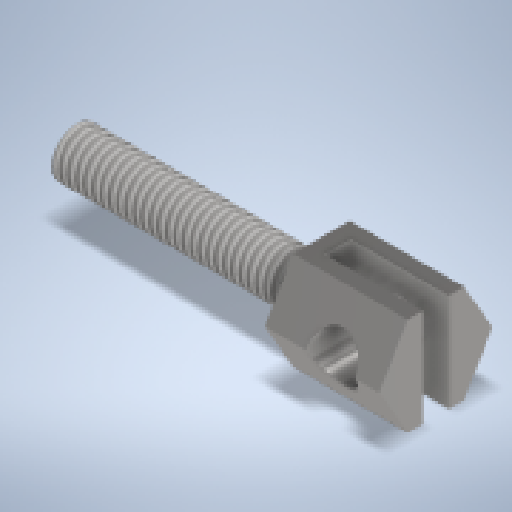
# Autodesk Inventor part: CompressionRollerArmActuatorScrew
Saved by Autodesk Inventor 2025 (Build 290162000, 162)
## iProperties
Created: 2024-08-19
Part Number: CompressionRollerArmActuatorScrew
Material: Steel, Alloy
Document SubType Name: Modeling
Designer: hello
Density: 7.73 g/cm^3
Appearance: Semi-Polished
Author: hello
Autodesk Inventor part; units mm, degrees
ref_plane "YZ Plane" through (0, 0, 0) normal (1, 0, 0) x (0, 1, 0)
ref_plane "XZ Plane" through (0, 0, 0) normal (0, 1, 0) x (-1, 0, 0)
ref_plane "XY Plane" through (0, 0, 0) normal (0, 0, 1) x (1, 0, 0)
sketch "Sketch1" plane through (0, 0, 0) normal (1, 0, 0) x (0, 1, 0)
  line L0 (3, -1.7321) -> (0, -3.4641)
  line L1 (0, -3.4641) -> (-3, -1.7321)
  line L2 (-3, -1.7321) -> (-3, 1.7321)
  line L3 (-3, 1.7321) -> (0, 3.4641)
  line L4 (0, 3.4641) -> (3, 1.7321)
  line L5 (3, 1.7321) -> (3, -1.7321)
  point P0 (0, 0)
  point P1 (0, 0)
  dimension "d0" = 6
  constraints: 12 end point, 1 coincident, 13 other
  measures "d0" distance between parallel lines of L2 L5
extrude "Extrusion1" add sketch "Sketch1" along normal blind 7
sketch "Sketch2" plane through (7, 0, 0) normal (1, 0, 0) x (0, 0, -1)
  line L0 (-0.8, 5) -> (0.8, 5)
  line L1 (0.8, 5) -> (0.8, -5)
  line L2 (0.8, -5) -> (-0.8, -5)
  line L3 (-0.8, -5) -> (-0.8, 5)
  line L4 (-0.8, 5) -> (0.8, -5) construction
  line L5 (0.8, 5) -> (-0.8, -5) construction
  point P0 (0, 0)
  dimension "d3" = 1.6
  dimension "d4" = 10
  constraints: 12 end point, 2 midpoint, 2 parallel, 1 horizontal, 1 perpendicular
  measures "d3" distance of L1.end L2.end
  measures "d4" distance of L0.end L1.end
extrude "Extrusion2" cut sketch "Sketch2" against normal blind 6
sketch "Sketch3" plane through (0, 0, 0) normal (-1, 0, 0) x (0, 0, 1)
  circle A0 centre (0, 0) radius 1.5
  dimension "d7" = 3
  constraints: 1 centre point, 1 coincident
  measures "d7" diameter of A0
extrude "Extrusion3" add sketch "Sketch3" along normal blind 15
thread "Thread1" size "M3x0.5" class "6g" standard "ANSI Metric M Profile" full length
sketch "Sketch4" plane through (7, -3, 0.8) normal (0, 0, -1) x (-1, 0, 0)
  line L0 (0, 6) -> (6, 6) projected
  line L1 (0, 0) -> (0, 6) projected
  line L2 (6, 0) -> (0, 0) projected
  line L3 (6, 0) -> (6, 6) projected
  line L4 (0, 0) -> (0, 6) projected
  circle A0 centre (3, 3) radius 1.5
  point P0 (7, 3)
  point P1 (3, 6)
  point P2 (0, 3)
  dimension "d12" = 3
  constraints: 2 midpoint, 1 centre point, 1 coincident, 1 horizontal alignment, 1 vertical alignment
  measures "d12" diameter of A0
extrude "Extrusion4" cut sketch "Sketch4" along normal through all both and the other way through all contours A0
body "Solid1"
